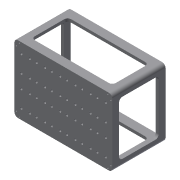
# Autodesk Inventor part: 05_Omniscope_base_v1
Saved by Autodesk Inventor 2019 (Build 230136000, 136)
## iProperties
Created: 2021-09-23
Part Number: 05_Omniscope_base_v1
Material: Generisch
Document SubType Name: Modeling
Designer: Muriel
Density: 1 g/cm^3
Appearance: Vorgabe
Author: Muriel
Autodesk Inventor part; units mm, degrees
(part 1 of 2)
ref_plane "YZ Plane" through (0, 0, 0) normal (1, 0, 0) x (0, 1, 0)
ref_plane "XZ Plane" through (0, 0, 0) normal (0, 1, 0) x (-1, 0, 0)
ref_plane "XY Plane" through (0, 0, 0) normal (0, 0, 1) x (1, 0, 0)
ref_plane "Arbeitsebene1" through (0, 0, 0) normal (0, 0, 1) x (1, 0, 0)
sketch "Skizze1" plane through (0, 0, 0) normal (0, 0, 1) x (1, 0, 0)
  arc A0 (4.5124, -17.9) -> (2.1124, -17.9) centre (3.3124, -16.3) ccw construction
  line L0 (4.5124, -17.9) -> (5.3124, -17.9) construction
  line L1 (5.3124, -17.9) -> (6.3124, -16.9) construction
  line L2 (6.3124, -16.9) -> (6.3124, 16.9) construction
  line L3 (6.3124, 16.9) -> (5.3124, 17.9) construction
  line L4 (5.3124, 17.9) -> (4.5124, 17.9) construction
  arc A1 (2.1124, 17.9) -> (4.5124, 17.9) centre (3.3124, 16.3) ccw construction
  line L5 (2.1124, 17.9) -> (-7.2876, 17.9) construction
  arc A2 (-9.6876, 17.9) -> (-7.2876, 17.9) centre (-8.4876, 16.3) ccw construction
  line L6 (-9.6876, 17.9) -> (-10.4876, 17.9) construction
  line L7 (-10.4876, 17.9) -> (-11.4876, 16.9) construction
  line L8 (-11.4876, 16.9) -> (-11.4876, -16.9) construction
  line L9 (-11.4876, -16.9) -> (-10.4876, -17.9) construction
  line L10 (-10.4876, -17.9) -> (-9.6876, -17.9) construction
  arc A3 (-7.2876, -17.9) -> (-9.6876, -17.9) centre (-8.4876, -16.3) ccw construction
  line L11 (-7.2876, -17.9) -> (2.1124, -17.9) construction
  circle A4 centre (-7.5876, -10) radius 2.45 construction
  circle A5 centre (2.4124, 10) radius 2.45 construction
  circle A6 centre (2.4124, -10) radius 2.45 construction
  circle A7 centre (-7.5876, 10) radius 2.45 construction
  line L12 (-5.4042, -5.4399) -> (-5.4042, -5.8455) construction
  line L13 (-5.4042, -5.8455) -> (-7.5626, -5.8455) construction
  line L14 (-7.5626, -5.8455) -> (-7.5626, -5.3491) construction
  spline S0 degree 2 poles (-7.5626, -5.3491) (-7.33, -5.1308) (-6.9159, -4.7252) (-6.7174, -4.5068) knots 0 0 0 1 2 2 2 construction
  spline S1 degree 2 poles (-6.7174, -4.5068) (-6.3174, -4.0671) (-6.0253, -3.5396) (-6.0253, -3.2588) knots 0 0 0 1 2 2 2 construction
  spline S2 degree 2 poles (-6.0253, -3.2588) (-6.0253, -3.1113) (-6.1161, -2.8901) (-6.1983, -2.8192) knots 0 0 0 1 2 2 2 construction
  spline S3 degree 2 poles (-6.1983, -2.8192) (-6.2806, -2.7483) (-6.4961, -2.6774) (-6.6266, -2.6774) knots 0 0 0 1 2 2 2 construction
  spline S4 degree 2 poles (-6.6266, -2.6774) (-6.7514, -2.6774) (-7.0067, -2.7397) (-7.123, -2.788) knots 0 0 0 1 2 2 2 construction
  spline S5 degree 2 poles (-7.123, -2.788) (-7.2222, -2.8277) (-7.4066, -2.9411) (-7.4633, -2.9808) knots 0 0 0 1 2 2 2 construction
  line L15 (-7.4633, -2.9808) -> (-7.4888, -2.9808) construction
  line L16 (-7.4888, -2.9808) -> (-7.4888, -2.4816) construction
  spline S6 degree 2 poles (-7.4888, -2.4816) (-7.3442, -2.4107) (-6.8251, -2.2718) (-6.5926, -2.2718) knots 0 0 0 1 2 2 2 construction
  spline S7 degree 2 poles (-6.5926, -2.2718) (-6.1019, -2.2718) (-5.5488, -2.7908) (-5.5488, -3.2333) knots 0 0 0 1 2 2 2 construction
  spline S8 degree 2 poles (-5.5488, -3.2333) (-5.5488, -3.4403) (-5.6452, -3.7863) (-5.7303, -3.9338) knots 0 0 0 1 2 2 2 construction
  spline S9 degree 2 poles (-5.7303, -3.9338) (-5.8154, -4.087) (-6.0622, -4.3876) (-6.1983, -4.5323) knots 0 0 0 1 2 2 2 construction
  spline S10 degree 2 poles (-6.1983, -4.5323) (-6.4195, -4.7734) (-6.9613, -5.2896) (-7.123, -5.4399) knots 0 0 0 1 2 2 2 construction
  line L17 (-7.123, -5.4399) -> (-5.4042, -5.4399) construction
  line L18 (1.5472, -2.3689) -> (1.5472, -5.8689) construction
  line L19 (1.5472, -5.8689) -> (1.0253, -5.8689) construction
  line L20 (1.0253, -5.8689) -> (-0.5233, -2.8511) construction
  line L21 (-0.5233, -2.8511) -> (-0.5233, -5.8689) construction
  line L22 (-0.5233, -5.8689) -> (-0.9572, -5.8689) construction
  line L23 (-0.9572, -5.8689) -> (-0.9572, -2.3689) construction
  line L24 (-0.9572, -2.3689) -> (-0.2964, -2.3689) construction
  line L25 (-0.2964, -2.3689) -> (1.1133, -5.14) construction
  line L26 (1.1133, -5.14) -> (1.1133, -2.3689) construction
  line L27 (1.1133, -2.3689) -> (1.5472, -2.3689) construction
  line L28 (3.2085, 3.1097) -> (3.2085, 2.7523) construction
  line L29 (3.2085, 2.7523) -> (1.501, 2.7523) construction
  line L30 (1.501, 2.7523) -> (1.501, 3.1097) construction
  line L31 (1.501, 3.1097) -> (2.1364, 3.1097) construction
  line L32 (2.1364, 3.1097) -> (2.1364, 5.4553) construction
  line L33 (2.1364, 5.4553) -> (1.501, 5.4553) construction
  line L34 (1.501, 5.4553) -> (1.501, 5.7758) construction
  spline S11 degree 2 poles (1.501, 5.7758) (1.8612, 5.7758) (2.2016, 5.98) (2.2243, 6.2636) knots 0 0 0 1 2 2 2 construction
  line L35 (2.2243, 6.2636) -> (2.5873, 6.2636) construction
  line L36 (2.5873, 6.2636) -> (2.5873, 3.1097) construction
  line L37 (2.5873, 3.1097) -> (3.2085, 3.1097) construction
  line L38 (-5.0676, 6.369) -> (-4.5939, 6.369) construction
  line L39 (-4.5939, 6.369) -> (-5.7994, 2.869) construction
  line L40 (-5.7994, 2.869) -> (-6.3014, 2.869) construction
  line L41 (-6.3014, 2.869) -> (-7.5068, 6.369) construction
  line L42 (-7.5068, 6.369) -> (-7.0076, 6.369) construction
  line L43 (-7.0076, 6.369) -> (-6.0376, 3.4618) construction
  line L44 (-6.0376, 3.4618) -> (-5.0676, 6.369) construction
  spline S12 degree 2 poles (-8.0968, 4.8261) (-7.9238, 4.6956) (-7.7366, 4.2985) (-7.7366, 3.9809) knots 0 0 0 1 2 2 2 construction
  spline S13 degree 2 poles (-7.7366, 3.9809) (-7.7366, 3.7284) (-7.8982, 3.2973) (-8.0457, 3.1385) knots 0 0 0 1 2 2 2 construction
  spline S14 degree 2 poles (-8.0457, 3.1385) (-8.1932, 2.9796) (-8.6328, 2.7953) (-8.9051, 2.7953) knots 0 0 0 1 2 2 2 construction
  spline S15 degree 2 poles (-8.9051, 2.7953) (-9.1547, 2.7953) (-9.6426, 2.9059) (-9.8212, 2.9938) knots 0 0 0 1 2 2 2 construction
  line L45 (-9.8212, 2.9938) -> (-9.8212, 3.4902) construction
  line L46 (-9.8212, 3.4902) -> (-9.7872, 3.4902) construction
  spline S16 degree 2 poles (-9.7872, 3.4902) (-9.7333, 3.4505) (-9.5319, 3.3484) (-9.41, 3.303) knots 0 0 0 1 2 2 2 construction
  spline S17 degree 2 poles (-9.41, 3.303) (-9.271, 3.2548) (-9.0413, 3.2009) (-8.8966, 3.2009) knots 0 0 0 1 2 2 2 construction
  spline S18 degree 2 poles (-8.8966, 3.2009) (-8.7548, 3.2009) (-8.4882, 3.303) (-8.3917, 3.4136) knots 0 0 0 1 2 2 2 construction
  spline S19 degree 2 poles (-8.3917, 3.4136) (-8.3038, 3.5185) (-8.2131, 3.7965) (-8.2131, 3.9837) knots 0 0 0 1 2 2 2 construction
  spline S20 degree 2 poles (-8.2131, 3.9837) (-8.2131, 4.1709) (-8.3152, 4.4091) (-8.4116, 4.4886) knots 0 0 0 1 2 2 2 construction
  spline S21 degree 2 poles (-8.4116, 4.4886) (-8.5109, 4.5765) (-8.8058, 4.6502) (-8.9845, 4.6502) knots 0 0 0 1 2 2 2 construction
  spline S22 degree 2 poles (-8.9845, 4.6502) (-9.1774, 4.6502) (-9.5603, 4.5907) (-9.6766, 4.5651) knots 0 0 0 1 2 2 2 construction
  line L47 (-9.6766, 4.5651) -> (-9.6766, 6.369) construction
  line L48 (-9.6766, 6.369) -> (-7.7564, 6.369) construction
  line L49 (-7.7564, 6.369) -> (-7.7564, 5.9578) construction
  line L50 (-7.7564, 5.9578) -> (-9.2256, 5.9578) construction
  line L51 (-9.2256, 5.9578) -> (-9.2256, 5.0246) construction
  spline S23 degree 2 poles (-9.2256, 5.0246) (-9.1405, 5.036) (-8.976, 5.0445) (-8.908, 5.0445) knots 0 0 0 1 2 2 2 construction
  spline S24 degree 2 poles (-8.908, 5.0445) (-8.6385, 5.0445) (-8.267, 4.9565) (-8.0968, 4.8261) knots 0 0 0 1 2 2 2 construction
  line L52 (-0.2036, 2.7523) -> (-0.6687, 2.7523) construction
  line L53 (-0.6687, 2.7523) -> (-0.6687, 5.8382) construction
  line L54 (-0.6687, 5.8382) -> (-1.843, 5.8382) construction
  line L55 (-1.843, 5.8382) -> (-1.843, 6.2523) construction
  line L56 (-1.843, 6.2523) -> (0.9706, 6.2523) construction
  line L57 (0.9706, 6.2523) -> (0.9706, 5.8382) construction
  line L58 (0.9706, 5.8382) -> (-0.2036, 5.8382) construction
  line L59 (-0.2036, 5.8382) -> (-0.2036, 2.7523) construction
  spline S25 degree 2 poles (-2.0577, -5.8349) (-2.2307, -5.886) (-2.5087, -5.937) (-2.7044, -5.937) knots 0 0 0 1 2 2 2 construction
  spline S26 degree 2 poles (-2.7044, -5.937) (-3.076, -5.937) (-3.6914, -5.7101) (-3.9127, -5.4804) knots 0 0 0 1 2 2 2 construction
  spline S27 degree 2 poles (-3.9127, -5.4804) (-4.1339, -5.2478) (-4.3693, -4.5614) (-4.3693, -4.1161) knots 0 0 0 1 2 2 2 construction
  spline S28 degree 2 poles (-4.3693, -4.1161) (-4.3693, -3.6935) (-4.1311, -3.0241) (-3.9098, -2.7859) knots 0 0 0 1 2 2 2 construction
  spline S29 degree 2 poles (-3.9098, -2.7859) (-3.6971, -2.5561) (-3.0731, -2.3065) (-2.7016, -2.3065) knots 0 0 0 1 2 2 2 construction
  spline S30 degree 2 poles (-2.7016, -2.3065) (-2.5229, -2.3065) (-2.1995, -2.3576) (-2.052, -2.403) knots 0 0 0 1 2 2 2 construction
  spline S31 degree 2 poles (-2.052, -2.403) (-1.9329, -2.437) (-1.6436, -2.5618) (-1.5557, -2.6072) knots 0 0 0 1 2 2 2 construction
  line L60 (-1.5557, -2.6072) -> (-1.5557, -3.1688) construction
  line L61 (-1.5557, -3.1688) -> (-1.5954, -3.1688) construction
  spline S32 degree 2 poles (-1.5954, -3.1688) (-1.6833, -3.0922) (-1.8677, -2.9532) (-2.0379, -2.8738) knots 0 0 0 1 2 2 2 construction
  spline S33 degree 2 poles (-2.0379, -2.8738) (-2.1797, -2.8029) (-2.5456, -2.7093) (-2.7554, -2.7093) knots 0 0 0 1 2 2 2 construction
  spline S34 degree 2 poles (-2.7554, -2.7093) (-3.2603, -2.7093) (-3.8843, -3.4694) (-3.8843, -4.1019) knots 0 0 0 1 2 2 2 construction
  spline S35 degree 2 poles (-3.8843, -4.1019) (-3.8843, -4.4536) (-3.7198, -4.9812) (-3.5638, -5.1627) knots 0 0 0 1 2 2 2 construction
  spline S36 degree 2 poles (-3.5638, -5.1627) (-3.4135, -5.3442) (-2.988, -5.5343) (-2.7214, -5.5343) knots 0 0 0 1 2 2 2 construction
  spline S37 degree 2 poles (-2.7214, -5.5343) (-2.5257, -5.5343) (-2.1343, -5.4775) (-2.001, -5.4208) knots 0 0 0 1 2 2 2 construction
  line L62 (-2.001, -5.4208) -> (-2.001, -4.516) construction
  line L63 (-2.001, -4.516) -> (-2.8122, -4.516) construction
  line L64 (-2.8122, -4.516) -> (-2.8122, -4.1076) construction
  line L65 (-2.8122, -4.1076) -> (-1.5415, -4.1076) construction
  line L66 (-1.5415, -4.1076) -> (-1.5415, -5.6364) construction
  spline S38 degree 2 poles (-1.5415, -5.6364) (-1.6294, -5.6761) (-1.9301, -5.798) (-2.0577, -5.8349) knots 0 0 0 1 2 2 2 construction
  spline S39 degree 2 poles (4.307, -2.6469) (4.6445, -2.871) (5.016, -3.6112) (5.016, -4.1218) knots 0 0 0 1 2 2 2 construction
  spline S40 degree 2 poles (5.016, -4.1218) (5.016, -4.6011) (4.6275, -5.3726) (4.3013, -5.5881) knots 0 0 0 1 2 2 2 construction
  spline S41 degree 2 poles (4.3013, -5.5881) (4.0347, -5.7555) (3.4873, -5.8689) (3.0618, -5.8689) knots 0 0 0 1 2 2 2 construction
  line L67 (3.0618, -5.8689) -> (2.2563, -5.8689) construction
  line L68 (2.2563, -5.8689) -> (2.2563, -2.3689) construction
  line L69 (2.2563, -2.3689) -> (3.0533, -2.3689) construction
  spline S42 degree 2 poles (3.0533, -2.3689) (3.5468, -2.3689) (4.1084, -2.5164) (4.307, -2.6469) knots 0 0 0 1 2 2 2 construction
  line L70 (-8.9921, -5.8455) -> (-9.4572, -5.8455) construction
  line L71 (-9.4572, -5.8455) -> (-9.4572, -2.7596) construction
  line L72 (-9.4572, -2.7596) -> (-10.6315, -2.7596) construction
  line L73 (-10.6315, -2.7596) -> (-10.6315, -2.3455) construction
  line L74 (-10.6315, -2.3455) -> (-7.8178, -2.3455) construction
  line L75 (-7.8178, -2.3455) -> (-7.8178, -2.7596) construction
  line L76 (-7.8178, -2.7596) -> (-8.9921, -2.7596) construction
  line L77 (-8.9921, -2.7596) -> (-8.9921, -5.8455) construction
  arc A8 (4.5124, -53.9) -> (2.1124, -53.9) centre (3.3124, -52.3) ccw construction
  line L78 (4.5124, -53.9) -> (5.3124, -53.9) construction
  line L79 (5.3124, -53.9) -> (6.3124, -52.9) construction
  line L80 (6.3124, -52.9) -> (6.3124, -19.1) construction
  line L81 (6.3124, -19.1) -> (5.3124, -18.1) construction
  line L82 (5.3124, -18.1) -> (4.5124, -18.1) construction
  arc A9 (2.1124, -18.1) -> (4.5124, -18.1) centre (3.3124, -19.7) ccw construction
  line L83 (2.1124, -18.1) -> (-7.2876, -18.1) construction
  arc A10 (-9.6876, -18.1) -> (-7.2876, -18.1) centre (-8.4876, -19.7) ccw construction
  line L84 (-9.6876, -18.1) -> (-10.4876, -18.1) construction
  line L85 (-10.4876, -18.1) -> (-11.4876, -19.1) construction
  line L86 (-11.4876, -19.1) -> (-11.4876, -52.9) construction
  line L87 (-11.4876, -52.9) -> (-10.4876, -53.9) construction
  line L88 (-10.4876, -53.9) -> (-9.6876, -53.9) construction
  arc A11 (-7.2876, -53.9) -> (-9.6876, -53.9) centre (-8.4876, -52.3) ccw construction
  line L89 (-7.2876, -53.9) -> (2.1124, -53.9) construction
  circle A12 centre (-7.5876, -46) radius 2.45 construction
  circle A13 centre (2.4124, -26) radius 2.45 construction
  circle A14 centre (2.4124, -46) radius 2.45 construction
  circle A15 centre (-7.5876, -26) radius 2.45 construction
  line L90 (-5.4042, -41.4399) -> (-5.4042, -41.8455) construction
  line L91 (-5.4042, -41.8455) -> (-7.5626, -41.8455) construction
  line L92 (-7.5626, -41.8455) -> (-7.5626, -41.3491) construction
  spline S43 degree 2 poles (-7.5626, -41.3491) (-7.33, -41.1308) (-6.9159, -40.7252) (-6.7174, -40.5068) knots 0 0 0 1 2 2 2 construction
  spline S44 degree 2 poles (-6.7174, -40.5068) (-6.3174, -40.0671) (-6.0253, -39.5396) (-6.0253, -39.2588) knots 0 0 0 1 2 2 2 construction
  spline S45 degree 2 poles (-6.0253, -39.2588) (-6.0253, -39.1113) (-6.1161, -38.8901) (-6.1983, -38.8192) knots 0 0 0 1 2 2 2 construction
  spline S46 degree 2 poles (-6.1983, -38.8192) (-6.2806, -38.7483) (-6.4961, -38.6774) (-6.6266, -38.6774) knots 0 0 0 1 2 2 2 construction
  spline S47 degree 2 poles (-6.6266, -38.6774) (-6.7514, -38.6774) (-7.0067, -38.7397) (-7.123, -38.788) knots 0 0 0 1 2 2 2 construction
  spline S48 degree 2 poles (-7.123, -38.788) (-7.2222, -38.8277) (-7.4066, -38.9411) (-7.4633, -38.9808) knots 0 0 0 1 2 2 2 construction
  line L93 (-7.4633, -38.9808) -> (-7.4888, -38.9808) construction
  line L94 (-7.4888, -38.9808) -> (-7.4888, -38.4816) construction
  spline S49 degree 2 poles (-7.4888, -38.4816) (-7.3442, -38.4107) (-6.8251, -38.2718) (-6.5926, -38.2718) knots 0 0 0 1 2 2 2 construction
  spline S50 degree 2 poles (-6.5926, -38.2718) (-6.1019, -38.2718) (-5.5488, -38.7908) (-5.5488, -39.2333) knots 0 0 0 1 2 2 2 construction
  spline S51 degree 2 poles (-5.5488, -39.2333) (-5.5488, -39.4403) (-5.6452, -39.7863) (-5.7303, -39.9338) knots 0 0 0 1 2 2 2 construction
  spline S52 degree 2 poles (-5.7303, -39.9338) (-5.8154, -40.087) (-6.0622, -40.3876) (-6.1983, -40.5323) knots 0 0 0 1 2 2 2 construction
  spline S53 degree 2 poles (-6.1983, -40.5323) (-6.4195, -40.7734) (-6.9613, -41.2896) (-7.123, -41.4399) knots 0 0 0 1 2 2 2 construction
  line L95 (-7.123, -41.4399) -> (-5.4042, -41.4399) construction
  line L96 (1.5472, -38.3689) -> (1.5472, -41.8689) construction
  line L97 (1.5472, -41.8689) -> (1.0253, -41.8689) construction
  line L98 (1.0253, -41.8689) -> (-0.5233, -38.8511) construction
  line L99 (-0.5233, -38.8511) -> (-0.5233, -41.8689) construction
  line L100 (-0.5233, -41.8689) -> (-0.9572, -41.8689) construction
  line L101 (-0.9572, -41.8689) -> (-0.9572, -38.3689) construction
  line L102 (-0.9572, -38.3689) -> (-0.2964, -38.3689) construction
  line L103 (-0.2964, -38.3689) -> (1.1133, -41.14) construction
  line L104 (1.1133, -41.14) -> (1.1133, -38.3689) construction
  line L105 (1.1133, -38.3689) -> (1.5472, -38.3689) construction
  line L106 (3.2085, -32.8903) -> (3.2085, -33.2477) construction
  line L107 (3.2085, -33.2477) -> (1.501, -33.2477) construction
  line L108 (1.501, -33.2477) -> (1.501, -32.8903) construction
  line L109 (1.501, -32.8903) -> (2.1364, -32.8903) construction
  line L110 (2.1364, -32.8903) -> (2.1364, -30.5447) construction
  line L111 (2.1364, -30.5447) -> (1.501, -30.5447) construction
  line L112 (1.501, -30.5447) -> (1.501, -30.2242) construction
  spline S54 degree 2 poles (1.501, -30.2242) (1.8612, -30.2242) (2.2016, -30.02) (2.2243, -29.7364) knots 0 0 0 1 2 2 2 construction
  line L113 (2.2243, -29.7364) -> (2.5873, -29.7364) construction
  line L114 (2.5873, -29.7364) -> (2.5873, -32.8903) construction
  line L115 (2.5873, -32.8903) -> (3.2085, -32.8903) construction
  line L116 (-5.0676, -29.631) -> (-4.5939, -29.631) construction
  line L117 (-4.5939, -29.631) -> (-5.7994, -33.131) construction
  line L118 (-5.7994, -33.131) -> (-6.3014, -33.131) construction
  line L119 (-6.3014, -33.131) -> (-7.5068, -29.631) construction
  line L120 (-7.5068, -29.631) -> (-7.0076, -29.631) construction
  line L121 (-7.0076, -29.631) -> (-6.0376, -32.5382) construction
  line L122 (-6.0376, -32.5382) -> (-5.0676, -29.631) construction
  spline S55 degree 2 poles (-8.0968, -31.1739) (-7.9238, -31.3044) (-7.7366, -31.7015) (-7.7366, -32.0191) knots 0 0 0 1 2 2 2 construction
  spline S56 degree 2 poles (-7.7366, -32.0191) (-7.7366, -32.2716) (-7.8982, -32.7027) (-8.0457, -32.8615) knots 0 0 0 1 2 2 2 construction
  spline S57 degree 2 poles (-8.0457, -32.8615) (-8.1932, -33.0204) (-8.6328, -33.2047) (-8.9051, -33.2047) knots 0 0 0 1 2 2 2 construction
  spline S58 degree 2 poles (-8.9051, -33.2047) (-9.1547, -33.2047) (-9.6426, -33.0941) (-9.8212, -33.0062) knots 0 0 0 1 2 2 2 construction
  line L123 (-9.8212, -33.0062) -> (-9.8212, -32.5098) construction
  line L124 (-9.8212, -32.5098) -> (-9.7872, -32.5098) construction
  spline S59 degree 2 poles (-9.7872, -32.5098) (-9.7333, -32.5495) (-9.5319, -32.6516) (-9.41, -32.697) knots 0 0 0 1 2 2 2 construction
  spline S60 degree 2 poles (-9.41, -32.697) (-9.271, -32.7452) (-9.0413, -32.7991) (-8.8966, -32.7991) knots 0 0 0 1 2 2 2 construction
  spline S61 degree 2 poles (-8.8966, -32.7991) (-8.7548, -32.7991) (-8.4882, -32.697) (-8.3917, -32.5864) knots 0 0 0 1 2 2 2 construction
  spline S62 degree 2 poles (-8.3917, -32.5864) (-8.3038, -32.4815) (-8.2131, -32.2035) (-8.2131, -32.0163) knots 0 0 0 1 2 2 2 construction
  spline S63 degree 2 poles (-8.2131, -32.0163) (-8.2131, -31.8291) (-8.3152, -31.5909) (-8.4116, -31.5114) knots 0 0 0 1 2 2 2 construction
  spline S64 degree 2 poles (-8.4116, -31.5114) (-8.5109, -31.4235) (-8.8058, -31.3498) (-8.9845, -31.3498) knots 0 0 0 1 2 2 2 construction
  spline S65 degree 2 poles (-8.9845, -31.3498) (-9.1774, -31.3498) (-9.5603, -31.4093) (-9.6766, -31.4349) knots 0 0 0 1 2 2 2 construction
  line L125 (-9.6766, -31.4349) -> (-9.6766, -29.631) construction
  line L126 (-9.6766, -29.631) -> (-7.7564, -29.631) construction
  line L127 (-7.7564, -29.631) -> (-7.7564, -30.0422) construction
  line L128 (-7.7564, -30.0422) -> (-9.2256, -30.0422) construction
  line L129 (-9.2256, -30.0422) -> (-9.2256, -30.9754) construction
  spline S66 degree 2 poles (-9.2256, -30.9754) (-9.1405, -30.964) (-8.976, -30.9555) (-8.908, -30.9555) knots 0 0 0 1 2 2 2 construction
  spline S67 degree 2 poles (-8.908, -30.9555) (-8.6385, -30.9555) (-8.267, -31.0435) (-8.0968, -31.1739) knots 0 0 0 1 2 2 2 construction
  line L130 (-0.2036, -33.2477) -> (-0.6687, -33.2477) construction
  line L131 (-0.6687, -33.2477) -> (-0.6687, -30.1618) construction
  line L132 (-0.6687, -30.1618) -> (-1.843, -30.1618) construction
  line L133 (-1.843, -30.1618) -> (-1.843, -29.7477) construction
  line L134 (-1.843, -29.7477) -> (0.9706, -29.7477) construction
  line L135 (0.9706, -29.7477) -> (0.9706, -30.1618) construction
  line L136 (0.9706, -30.1618) -> (-0.2036, -30.1618) construction
  line L137 (-0.2036, -30.1618) -> (-0.2036, -33.2477) construction
  spline S68 degree 2 poles (-2.0577, -41.8349) (-2.2307, -41.886) (-2.5087, -41.937) (-2.7044, -41.937) knots 0 0 0 1 2 2 2 construction
  spline S69 degree 2 poles (-2.7044, -41.937) (-3.076, -41.937) (-3.6914, -41.7101) (-3.9127, -41.4804) knots 0 0 0 1 2 2 2 construction
  spline S70 degree 2 poles (-3.9127, -41.4804) (-4.1339, -41.2478) (-4.3693, -40.5614) (-4.3693, -40.1161) knots 0 0 0 1 2 2 2 construction
  spline S71 degree 2 poles (-4.3693, -40.1161) (-4.3693, -39.6935) (-4.1311, -39.0241) (-3.9098, -38.7859) knots 0 0 0 1 2 2 2 construction
  spline S72 degree 2 poles (-3.9098, -38.7859) (-3.6971, -38.5561) (-3.0731, -38.3065) (-2.7016, -38.3065) knots 0 0 0 1 2 2 2 construction
  spline S73 degree 2 poles (-2.7016, -38.3065) (-2.5229, -38.3065) (-2.1995, -38.3576) (-2.052, -38.403) knots 0 0 0 1 2 2 2 construction
  spline S74 degree 2 poles (-2.052, -38.403) (-1.9329, -38.437) (-1.6436, -38.5618) (-1.5557, -38.6072) knots 0 0 0 1 2 2 2 construction
  line L138 (-1.5557, -38.6072) -> (-1.5557, -39.1688) construction
  line L139 (-1.5557, -39.1688) -> (-1.5954, -39.1688) construction
  spline S75 degree 2 poles (-1.5954, -39.1688) (-1.6833, -39.0922) (-1.8677, -38.9532) (-2.0379, -38.8738) knots 0 0 0 1 2 2 2 construction
  spline S76 degree 2 poles (-2.0379, -38.8738) (-2.1797, -38.8029) (-2.5456, -38.7093) (-2.7554, -38.7093) knots 0 0 0 1 2 2 2 construction
  spline S77 degree 2 poles (-2.7554, -38.7093) (-3.2603, -38.7093) (-3.8843, -39.4694) (-3.8843, -40.1019) knots 0 0 0 1 2 2 2 construction
  spline S78 degree 2 poles (-3.8843, -40.1019) (-3.8843, -40.4536) (-3.7198, -40.9812) (-3.5638, -41.1627) knots 0 0 0 1 2 2 2 construction
  spline S79 degree 2 poles (-3.5638, -41.1627) (-3.4135, -41.3442) (-2.988, -41.5343) (-2.7214, -41.5343) knots 0 0 0 1 2 2 2 construction
  spline S80 degree 2 poles (-2.7214, -41.5343) (-2.5257, -41.5343) (-2.1343, -41.4775) (-2.001, -41.4208) knots 0 0 0 1 2 2 2 construction
  line L140 (-2.001, -41.4208) -> (-2.001, -40.516) construction
  line L141 (-2.001, -40.516) -> (-2.8122, -40.516) construction
  line L142 (-2.8122, -40.516) -> (-2.8122, -40.1076) construction
  line L143 (-2.8122, -40.1076) -> (-1.5415, -40.1076) construction
  line L144 (-1.5415, -40.1076) -> (-1.5415, -41.6364) construction
  spline S81 degree 2 poles (-1.5415, -41.6364) (-1.6294, -41.6761) (-1.9301, -41.798) (-2.0577, -41.8349) knots 0 0 0 1 2 2 2 construction
  spline S82 degree 2 poles (4.307, -38.6469) (4.6445, -38.871) (5.016, -39.6112) (5.016, -40.1218) knots 0 0 0 1 2 2 2 construction
  spline S83 degree 2 poles (5.016, -40.1218) (5.016, -40.6011) (4.6275, -41.3726) (4.3013, -41.5881) knots 0 0 0 1 2 2 2 construction
  spline S84 degree 2 poles (4.3013, -41.5881) (4.0347, -41.7555) (3.4873, -41.8689) (3.0618, -41.8689) knots 0 0 0 1 2 2 2 construction
  line L145 (3.0618, -41.8689) -> (2.2563, -41.8689) construction
  line L146 (2.2563, -41.8689) -> (2.2563, -38.3689) construction
  line L147 (2.2563, -38.3689) -> (3.0533, -38.3689) construction
  spline S85 degree 2 poles (3.0533, -38.3689) (3.5468, -38.3689) (4.1084, -38.5164) (4.307, -38.6469) knots 0 0 0 1 2 2 2 construction
  line L148 (-8.9921, -41.8455) -> (-9.4572, -41.8455) construction
  line L149 (-9.4572, -41.8455) -> (-9.4572, -38.7596) construction
  line L150 (-9.4572, -38.7596) -> (-10.6315, -38.7596) construction
  line L151 (-10.6315, -38.7596) -> (-10.6315, -38.3455) construction
  line L152 (-10.6315, -38.3455) -> (-7.8178, -38.3455) construction
  line L153 (-7.8178, -38.3455) -> (-7.8178, -38.7596) construction
  line L154 (-7.8178, -38.7596) -> (-8.9921, -38.7596) construction
  line L155 (-8.9921, -38.7596) -> (-8.9921, -41.8455) construction
  arc A16 (94.5124, -53.9) -> (92.1124, -53.9) centre (93.3124, -52.3) ccw construction
  line L156 (94.5124, -53.9) -> (95.3124, -53.9) construction
  line L157 (95.3124, -53.9) -> (96.3124, -52.9) construction
  line L158 (96.3124, -52.9) -> (96.3124, -19.1) construction
  line L159 (96.3124, -19.1) -> (95.3124, -18.1) construction
  line L160 (95.3124, -18.1) -> (94.5124, -18.1) construction
  arc A17 (92.1124, -18.1) -> (94.5124, -18.1) centre (93.3124, -19.7) ccw construction
  line L161 (92.1124, -18.1) -> (82.7124, -18.1) construction
  arc A18 (80.3124, -18.1) -> (82.7124, -18.1) centre (81.5124, -19.7) ccw construction
  line L162 (80.3124, -18.1) -> (79.5124, -18.1) construction
  line L163 (79.5124, -18.1) -> (78.5124, -19.1) construction
  line L164 (78.5124, -19.1) -> (78.5124, -52.9) construction
  line L165 (78.5124, -52.9) -> (79.5124, -53.9) construction
  line L166 (79.5124, -53.9) -> (80.3124, -53.9) construction
  arc A19 (82.7124, -53.9) -> (80.3124, -53.9) centre (81.5124, -52.3) ccw construction
  line L167 (82.7124, -53.9) -> (92.1124, -53.9) construction
  circle A20 centre (82.4124, -46) radius 2.45 construction
  circle A21 centre (92.4124, -26) radius 2.45 construction
  circle A22 centre (92.4124, -46) radius 2.45 construction
  circle A23 centre (82.4124, -26) radius 2.45 construction
  line L168 (84.5958, -41.4399) -> (84.5958, -41.8455) construction
  line L169 (84.5958, -41.8455) -> (82.4374, -41.8455) construction
  line L170 (82.4374, -41.8455) -> (82.4374, -41.3491) construction
  spline S86 degree 2 poles (82.4374, -41.3491) (82.67, -41.1308) (83.0841, -40.7252) (83.2826, -40.5068) knots 0 0 0 1 2 2 2 construction
  spline S87 degree 2 poles (83.2826, -40.5068) (83.6826, -40.0671) (83.9747, -39.5396) (83.9747, -39.2588) knots 0 0 0 1 2 2 2 construction
  spline S88 degree 2 poles (83.9747, -39.2588) (83.9747, -39.1113) (83.8839, -38.8901) (83.8017, -38.8192) knots 0 0 0 1 2 2 2 construction
  spline S89 degree 2 poles (83.8017, -38.8192) (83.7194, -38.7483) (83.5039, -38.6774) (83.3734, -38.6774) knots 0 0 0 1 2 2 2 construction
  spline S90 degree 2 poles (83.3734, -38.6774) (83.2486, -38.6774) (82.9933, -38.7397) (82.877, -38.788) knots 0 0 0 1 2 2 2 construction
  spline S91 degree 2 poles (82.877, -38.788) (82.7778, -38.8277) (82.5934, -38.9411) (82.5367, -38.9808) knots 0 0 0 1 2 2 2 construction
  line L171 (82.5367, -38.9808) -> (82.5112, -38.9808) construction
  line L172 (82.5112, -38.9808) -> (82.5112, -38.4816) construction
  spline S92 degree 2 poles (82.5112, -38.4816) (82.6558, -38.4107) (83.1749, -38.2718) (83.4074, -38.2718) knots 0 0 0 1 2 2 2 construction
  spline S93 degree 2 poles (83.4074, -38.2718) (83.8981, -38.2718) (84.4512, -38.7908) (84.4512, -39.2333) knots 0 0 0 1 2 2 2 construction
  spline S94 degree 2 poles (84.4512, -39.2333) (84.4512, -39.4403) (84.3548, -39.7863) (84.2697, -39.9338) knots 0 0 0 1 2 2 2 construction
  spline S95 degree 2 poles (84.2697, -39.9338) (84.1846, -40.087) (83.9378, -40.3876) (83.8017, -40.5323) knots 0 0 0 1 2 2 2 construction
  spline S96 degree 2 poles (83.8017, -40.5323) (83.5805, -40.7734) (83.0387, -41.2896) (82.877, -41.4399) knots 0 0 0 1 2 2 2 construction
  line L173 (82.877, -41.4399) -> (84.5958, -41.4399) construction
  line L174 (91.5472, -38.3689) -> (91.5472, -41.8689) construction
  line L175 (91.5472, -41.8689) -> (91.0253, -41.8689) construction
  line L176 (91.0253, -41.8689) -> (89.4767, -38.8511) construction
  line L177 (89.4767, -38.8511) -> (89.4767, -41.8689) construction
  line L178 (89.4767, -41.8689) -> (89.0428, -41.8689) construction
  line L179 (89.0428, -41.8689) -> (89.0428, -38.3689) construction
  line L180 (89.0428, -38.3689) -> (89.7036, -38.3689) construction
  line L181 (89.7036, -38.3689) -> (91.1133, -41.14) construction
  line L182 (91.1133, -41.14) -> (91.1133, -38.3689) construction
  line L183 (91.1133, -38.3689) -> (91.5472, -38.3689) construction
  line L184 (93.2085, -32.8903) -> (93.2085, -33.2477) construction
  line L185 (93.2085, -33.2477) -> (91.501, -33.2477) construction
  line L186 (91.501, -33.2477) -> (91.501, -32.8903) construction
  line L187 (91.501, -32.8903) -> (92.1364, -32.8903) construction
  line L188 (92.1364, -32.8903) -> (92.1364, -30.5447) construction
  line L189 (92.1364, -30.5447) -> (91.501, -30.5447) construction
  line L190 (91.501, -30.5447) -> (91.501, -30.2242) construction
  spline S97 degree 2 poles (91.501, -30.2242) (91.8612, -30.2242) (92.2016, -30.02) (92.2243, -29.7364) knots 0 0 0 1 2 2 2 construction
  line L191 (92.2243, -29.7364) -> (92.5873, -29.7364) construction
  line L192 (92.5873, -29.7364) -> (92.5873, -32.8903) construction
  line L193 (92.5873, -32.8903) -> (93.2085, -32.8903) construction
  line L194 (84.9324, -29.631) -> (85.4061, -29.631) construction
  line L195 (85.4061, -29.631) -> (84.2006, -33.131) construction
  line L196 (84.2006, -33.131) -> (83.6986, -33.131) construction
  line L197 (83.6986, -33.131) -> (82.4932, -29.631) construction
  line L198 (82.4932, -29.631) -> (82.9924, -29.631) construction
  line L199 (82.9924, -29.631) -> (83.9624, -32.5382) construction
  line L200 (83.9624, -32.5382) -> (84.9324, -29.631) construction
  spline S98 degree 2 poles (81.9032, -31.1739) (82.0762, -31.3044) (82.2634, -31.7015) (82.2634, -32.0191) knots 0 0 0 1 2 2 2 construction
  spline S99 degree 2 poles (82.2634, -32.0191) (82.2634, -32.2716) (82.1018, -32.7027) (81.9543, -32.8615) knots 0 0 0 1 2 2 2 construction
  spline S100 degree 2 poles (81.9543, -32.8615) (81.8068, -33.0204) (81.3672, -33.2047) (81.0949, -33.2047) knots 0 0 0 1 2 2 2 construction
  spline S101 degree 2 poles (81.0949, -33.2047) (80.8453, -33.2047) (80.3574, -33.0941) (80.1788, -33.0062) knots 0 0 0 1 2 2 2 construction
  line L201 (80.1788, -33.0062) -> (80.1788, -32.5098) construction
  line L202 (80.1788, -32.5098) -> (80.2128, -32.5098) construction
  spline S102 degree 2 poles (80.2128, -32.5098) (80.2667, -32.5495) (80.4681, -32.6516) (80.59, -32.697) knots 0 0 0 1 2 2 2 construction
  spline S103 degree 2 poles (80.59, -32.697) (80.729, -32.7452) (80.9587, -32.7991) (81.1034, -32.7991) knots 0 0 0 1 2 2 2 construction
  spline S104 degree 2 poles (81.1034, -32.7991) (81.2452, -32.7991) (81.5118, -32.697) (81.6083, -32.5864) knots 0 0 0 1 2 2 2 construction
  spline S105 degree 2 poles (81.6083, -32.5864) (81.6962, -32.4815) (81.7869, -32.2035) (81.7869, -32.0163) knots 0 0 0 1 2 2 2 construction
  spline S106 degree 2 poles (81.7869, -32.0163) (81.7869, -31.8291) (81.6848, -31.5909) (81.5884, -31.5114) knots 0 0 0 1 2 2 2 construction
  spline S107 degree 2 poles (81.5884, -31.5114) (81.4891, -31.4235) (81.1942, -31.3498) (81.0155, -31.3498) knots 0 0 0 1 2 2 2 construction
  spline S108 degree 2 poles (81.0155, -31.3498) (80.8226, -31.3498) (80.4397, -31.4093) (80.3234, -31.4349) knots 0 0 0 1 2 2 2 construction
  line L203 (80.3234, -31.4349) -> (80.3234, -29.631) construction
  line L204 (80.3234, -29.631) -> (82.2436, -29.631) construction
  line L205 (82.2436, -29.631) -> (82.2436, -30.0422) construction
  line L206 (82.2436, -30.0422) -> (80.7744, -30.0422) construction
  line L207 (80.7744, -30.0422) -> (80.7744, -30.9754) construction
  spline S109 degree 2 poles (80.7744, -30.9754) (80.8595, -30.964) (81.024, -30.9555) (81.092, -30.9555) knots 0 0 0 1 2 2 2 construction
  spline S110 degree 2 poles (81.092, -30.9555) (81.3615, -30.9555) (81.733, -31.0435) (81.9032, -31.1739) knots 0 0 0 1 2 2 2 construction
  line L208 (89.7964, -33.2477) -> (89.3313, -33.2477) construction
  line L209 (89.3313, -33.2477) -> (89.3313, -30.1618) construction
  line L210 (89.3313, -30.1618) -> (88.157, -30.1618) construction
  line L211 (88.157, -30.1618) -> (88.157, -29.7477) construction
  line L212 (88.157, -29.7477) -> (90.9706, -29.7477) construction
  line L213 (90.9706, -29.7477) -> (90.9706, -30.1618) construction
  line L214 (90.9706, -30.1618) -> (89.7964, -30.1618) construction
  line L215 (89.7964, -30.1618) -> (89.7964, -33.2477) construction
  spline S111 degree 2 poles (87.9423, -41.8349) (87.7693, -41.886) (87.4913, -41.937) (87.2956, -41.937) knots 0 0 0 1 2 2 2 construction
  spline S112 degree 2 poles (87.2956, -41.937) (86.924, -41.937) (86.3086, -41.7101) (86.0873, -41.4804) knots 0 0 0 1 2 2 2 construction
  spline S113 degree 2 poles (86.0873, -41.4804) (85.8661, -41.2478) (85.6307, -40.5614) (85.6307, -40.1161) knots 0 0 0 1 2 2 2 construction
  spline S114 degree 2 poles (85.6307, -40.1161) (85.6307, -39.6935) (85.8689, -39.0241) (86.0902, -38.7859) knots 0 0 0 1 2 2 2 construction
  spline S115 degree 2 poles (86.0902, -38.7859) (86.3029, -38.5561) (86.9269, -38.3065) (87.2984, -38.3065) knots 0 0 0 1 2 2 2 construction
  spline S116 degree 2 poles (87.2984, -38.3065) (87.4771, -38.3065) (87.8005, -38.3576) (87.948, -38.403) knots 0 0 0 1 2 2 2 construction
  spline S117 degree 2 poles (87.948, -38.403) (88.0671, -38.437) (88.3564, -38.5618) (88.4443, -38.6072) knots 0 0 0 1 2 2 2 construction
  line L216 (88.4443, -38.6072) -> (88.4443, -39.1688) construction
  line L217 (88.4443, -39.1688) -> (88.4046, -39.1688) construction
  spline S118 degree 2 poles (88.4046, -39.1688) (88.3167, -39.0922) (88.1323, -38.9532) (87.9621, -38.8738) knots 0 0 0 1 2 2 2 construction
  spline S119 degree 2 poles (87.9621, -38.8738) (87.8203, -38.8029) (87.4544, -38.7093) (87.2446, -38.7093) knots 0 0 0 1 2 2 2 construction
  spline S120 degree 2 poles (87.2446, -38.7093) (86.7397, -38.7093) (86.1157, -39.4694) (86.1157, -40.1019) knots 0 0 0 1 2 2 2 construction
  spline S121 degree 2 poles (86.1157, -40.1019) (86.1157, -40.4536) (86.2802, -40.9812) (86.4362, -41.1627) knots 0 0 0 1 2 2 2 construction
  spline S122 degree 2 poles (86.4362, -41.1627) (86.5865, -41.3442) (87.012, -41.5343) (87.2786, -41.5343) knots 0 0 0 1 2 2 2 construction
  spline S123 degree 2 poles (87.2786, -41.5343) (87.4743, -41.5343) (87.8657, -41.4775) (87.999, -41.4208) knots 0 0 0 1 2 2 2 construction
  line L218 (87.999, -41.4208) -> (87.999, -40.516) construction
  line L219 (87.999, -40.516) -> (87.1878, -40.516) construction
  line L220 (87.1878, -40.516) -> (87.1878, -40.1076) construction
  line L221 (87.1878, -40.1076) -> (88.4585, -40.1076) construction
  line L222 (88.4585, -40.1076) -> (88.4585, -41.6364) construction
  spline S124 degree 2 poles (88.4585, -41.6364) (88.3706, -41.6761) (88.0699, -41.798) (87.9423, -41.8349) knots 0 0 0 1 2 2 2 construction
  spline S125 degree 2 poles (94.307, -38.6469) (94.6445, -38.871) (95.016, -39.6112) (95.016, -40.1218) knots 0 0 0 1 2 2 2 construction
  spline S126 degree 2 poles (95.016, -40.1218) (95.016, -40.6011) (94.6275, -41.3726) (94.3013, -41.5881) knots 0 0 0 1 2 2 2 construction
  spline S127 degree 2 poles (94.3013, -41.5881) (94.0347, -41.7555) (93.4873, -41.8689) (93.0618, -41.8689) knots 0 0 0 1 2 2 2 construction
  line L223 (93.0618, -41.8689) -> (92.2563, -41.8689) construction
  line L224 (92.2563, -41.8689) -> (92.2563, -38.3689) construction
  line L225 (92.2563, -38.3689) -> (93.0533, -38.3689) construction
  spline S128 degree 2 poles (93.0533, -38.3689) (93.5468, -38.3689) (94.1084, -38.5164) (94.307, -38.6469) knots 0 0 0 1 2 2 2 construction
  line L226 (81.0079, -41.8455) -> (80.5428, -41.8455) construction
  line L227 (80.5428, -41.8455) -> (80.5428, -38.7596) construction
  line L228 (80.5428, -38.7596) -> (79.3685, -38.7596) construction
  line L229 (79.3685, -38.7596) -> (79.3685, -38.3455) construction
  line L230 (79.3685, -38.3455) -> (82.1822, -38.3455) construction
  line L231 (82.1822, -38.3455) -> (82.1822, -38.7596) construction
  line L232 (82.1822, -38.7596) -> (81.0079, -38.7596) construction
  line L233 (81.0079, -38.7596) -> (81.0079, -41.8455) construction
  arc A24 (94.5124, -17.9) -> (92.1124, -17.9) centre (93.3124, -16.3) ccw construction
  line L234 (94.5124, -17.9) -> (95.3124, -17.9) construction
  line L235 (95.3124, -17.9) -> (96.3124, -16.9) construction
  line L236 (96.3124, -16.9) -> (96.3124, 16.9) construction
  line L237 (96.3124, 16.9) -> (95.3124, 17.9) construction
  line L238 (95.3124, 17.9) -> (94.5124, 17.9) construction
  arc A25 (92.1124, 17.9) -> (94.5124, 17.9) centre (93.3124, 16.3) ccw construction
  line L239 (92.1124, 17.9) -> (82.7124, 17.9) construction
  arc A26 (80.3124, 17.9) -> (82.7124, 17.9) centre (81.5124, 16.3) ccw construction
  line L240 (80.3124, 17.9) -> (79.5124, 17.9) construction
  line L241 (79.5124, 17.9) -> (78.5124, 16.9) construction
  line L242 (78.5124, 16.9) -> (78.5124, -16.9) construction
  line L243 (78.5124, -16.9) -> (79.5124, -17.9) construction
  line L244 (79.5124, -17.9) -> (80.3124, -17.9) construction
  arc A27 (82.7124, -17.9) -> (80.3124, -17.9) centre (81.5124, -16.3) ccw construction
  line L245 (82.7124, -17.9) -> (92.1124, -17.9) construction
  circle A28 centre (82.4124, -10) radius 2.45 construction
  circle A29 centre (92.4124, 10) radius 2.45 construction
  circle A30 centre (92.4124, -10) radius 2.45 construction
  circle A31 centre (82.4124, 10) radius 2.45 construction
  line L246 (84.5958, -5.4399) -> (84.5958, -5.8455) construction
  line L247 (84.5958, -5.8455) -> (82.4374, -5.8455) construction
  line L248 (82.4374, -5.8455) -> (82.4374, -5.3491) construction
  spline S129 degree 2 poles (82.4374, -5.3491) (82.67, -5.1308) (83.0841, -4.7252) (83.2826, -4.5068) knots 0 0 0 1 2 2 2 construction
  spline S130 degree 2 poles (83.2826, -4.5068) (83.6826, -4.0671) (83.9747, -3.5396) (83.9747, -3.2588) knots 0 0 0 1 2 2 2 construction
  spline S131 degree 2 poles (83.9747, -3.2588) (83.9747, -3.1113) (83.8839, -2.8901) (83.8017, -2.8192) knots 0 0 0 1 2 2 2 construction
  spline S132 degree 2 poles (83.8017, -2.8192) (83.7194, -2.7483) (83.5039, -2.6774) (83.3734, -2.6774) knots 0 0 0 1 2 2 2 construction
  spline S133 degree 2 poles (83.3734, -2.6774) (83.2486, -2.6774) (82.9933, -2.7397) (82.877, -2.788) knots 0 0 0 1 2 2 2 construction
  spline S134 degree 2 poles (82.877, -2.788) (82.7778, -2.8277) (82.5934, -2.9411) (82.5367, -2.9808) knots 0 0 0 1 2 2 2 construction
  line L249 (82.5367, -2.9808) -> (82.5112, -2.9808) construction
  line L250 (82.5112, -2.9808) -> (82.5112, -2.4816) construction
  spline S135 degree 2 poles (82.5112, -2.4816) (82.6558, -2.4107) (83.1749, -2.2718) (83.4074, -2.2718) knots 0 0 0 1 2 2 2 construction
  spline S136 degree 2 poles (83.4074, -2.2718) (83.8981, -2.2718) (84.4512, -2.7908) (84.4512, -3.2333) knots 0 0 0 1 2 2 2 construction
  spline S137 degree 2 poles (84.4512, -3.2333) (84.4512, -3.4403) (84.3548, -3.7863) (84.2697, -3.9338) knots 0 0 0 1 2 2 2 construction
  spline S138 degree 2 poles (84.2697, -3.9338) (84.1846, -4.087) (83.9378, -4.3876) (83.8017, -4.5323) knots 0 0 0 1 2 2 2 construction
  spline S139 degree 2 poles (83.8017, -4.5323) (83.5805, -4.7734) (83.0387, -5.2896) (82.877, -5.4399) knots 0 0 0 1 2 2 2 construction
  line L251 (82.877, -5.4399) -> (84.5958, -5.4399) construction
  line L252 (91.5472, -2.3689) -> (91.5472, -5.8689) construction
  line L253 (91.5472, -5.8689) -> (91.0253, -5.8689) construction
  line L254 (91.0253, -5.8689) -> (89.4767, -2.8511) construction
  line L255 (89.4767, -2.8511) -> (89.4767, -5.8689) construction
  line L256 (89.4767, -5.8689) -> (89.0428, -5.8689) construction
  line L257 (89.0428, -5.8689) -> (89.0428, -2.3689) construction
  line L258 (89.0428, -2.3689) -> (89.7036, -2.3689) construction
  line L259 (89.7036, -2.3689) -> (91.1133, -5.14) construction
  line L260 (91.1133, -5.14) -> (91.1133, -2.3689) construction
  line L261 (91.1133, -2.3689) -> (91.5472, -2.3689) construction
  line L262 (93.2085, 3.1097) -> (93.2085, 2.7523) construction
  line L263 (93.2085, 2.7523) -> (91.501, 2.7523) construction
  line L264 (91.501, 2.7523) -> (91.501, 3.1097) construction
  line L265 (91.501, 3.1097) -> (92.1364, 3.1097) construction
  line L266 (92.1364, 3.1097) -> (92.1364, 5.4553) construction
  line L267 (92.1364, 5.4553) -> (91.501, 5.4553) construction
  line L268 (91.501, 5.4553) -> (91.501, 5.7758) construction
  spline S140 degree 2 poles (91.501, 5.7758) (91.8612, 5.7758) (92.2016, 5.98) (92.2243, 6.2636) knots 0 0 0 1 2 2 2 construction
  line L269 (92.2243, 6.2636) -> (92.5873, 6.2636) construction
  line L270 (92.5873, 6.2636) -> (92.5873, 3.1097) construction
  line L271 (92.5873, 3.1097) -> (93.2085, 3.1097) construction
  line L272 (84.9324, 6.369) -> (85.4061, 6.369) construction
  line L273 (85.4061, 6.369) -> (84.2006, 2.869) construction
  line L274 (84.2006, 2.869) -> (83.6986, 2.869) construction
  line L275 (83.6986, 2.869) -> (82.4932, 6.369) construction
  line L276 (82.4932, 6.369) -> (82.9924, 6.369) construction
  line L277 (82.9924, 6.369) -> (83.9624, 3.4618) construction
  line L278 (83.9624, 3.4618) -> (84.9324, 6.369) construction
  spline S141 degree 2 poles (81.9032, 4.8261) (82.0762, 4.6956) (82.2634, 4.2985) (82.2634, 3.9809) knots 0 0 0 1 2 2 2 construction
  spline S142 degree 2 poles (82.2634, 3.9809) (82.2634, 3.7284) (82.1018, 3.2973) (81.9543, 3.1385) knots 0 0 0 1 2 2 2 construction
  spline S143 degree 2 poles (81.9543, 3.1385) (81.8068, 2.9796) (81.3672, 2.7953) (81.0949, 2.7953) knots 0 0 0 1 2 2 2 construction
  spline S144 degree 2 poles (81.0949, 2.7953) (80.8453, 2.7953) (80.3574, 2.9059) (80.1788, 2.9938) knots 0 0 0 1 2 2 2 construction
  line L279 (80.1788, 2.9938) -> (80.1788, 3.4902) construction
  line L280 (80.1788, 3.4902) -> (80.2128, 3.4902) construction
  spline S145 degree 2 poles (80.2128, 3.4902) (80.2667, 3.4505) (80.4681, 3.3484) (80.59, 3.303) knots 0 0 0 1 2 2 2 construction
  spline S146 degree 2 poles (80.59, 3.303) (80.729, 3.2548) (80.9587, 3.2009) (81.1034, 3.2009) knots 0 0 0 1 2 2 2 construction
  spline S147 degree 2 poles (81.1034, 3.2009) (81.2452, 3.2009) (81.5118, 3.303) (81.6083, 3.4136) knots 0 0 0 1 2 2 2 construction
  spline S148 degree 2 poles (81.6083, 3.4136) (81.6962, 3.5185) (81.7869, 3.7965) (81.7869, 3.9837) knots 0 0 0 1 2 2 2 construction
  spline S149 degree 2 poles (81.7869, 3.9837) (81.7869, 4.1709) (81.6848, 4.4091) (81.5884, 4.4886) knots 0 0 0 1 2 2 2 construction
  spline S150 degree 2 poles (81.5884, 4.4886) (81.4891, 4.5765) (81.1942, 4.6502) (81.0155, 4.6502) knots 0 0 0 1 2 2 2 construction
  spline S151 degree 2 poles (81.0155, 4.6502) (80.8226, 4.6502) (80.4397, 4.5907) (80.3234, 4.5651) knots 0 0 0 1 2 2 2 construction
  line L281 (80.3234, 4.5651) -> (80.3234, 6.369) construction
  line L282 (80.3234, 6.369) -> (82.2436, 6.369) construction
  line L283 (82.2436, 6.369) -> (82.2436, 5.9578) construction
  line L284 (82.2436, 5.9578) -> (80.7744, 5.9578) construction
  line L285 (80.7744, 5.9578) -> (80.7744, 5.0246) construction
  spline S152 degree 2 poles (80.7744, 5.0246) (80.8595, 5.036) (81.024, 5.0445) (81.092, 5.0445) knots 0 0 0 1 2 2 2 construction
  spline S153 degree 2 poles (81.092, 5.0445) (81.3615, 5.0445) (81.733, 4.9565) (81.9032, 4.8261) knots 0 0 0 1 2 2 2 construction
  line L286 (89.7964, 2.7523) -> (89.3313, 2.7523) construction
  line L287 (89.3313, 2.7523) -> (89.3313, 5.8382) construction
  line L288 (89.3313, 5.8382) -> (88.157, 5.8382) construction
  line L289 (88.157, 5.8382) -> (88.157, 6.2523) construction
  line L290 (88.157, 6.2523) -> (90.9706, 6.2523) construction
  line L291 (90.9706, 6.2523) -> (90.9706, 5.8382) construction
  line L292 (90.9706, 5.8382) -> (89.7964, 5.8382) construction
  line L293 (89.7964, 5.8382) -> (89.7964, 2.7523) construction
  spline S154 degree 2 poles (87.9423, -5.8349) (87.7693, -5.886) (87.4913, -5.937) (87.2956, -5.937) knots 0 0 0 1 2 2 2 construction
  spline S155 degree 2 poles (87.2956, -5.937) (86.924, -5.937) (86.3086, -5.7101) (86.0873, -5.4804) knots 0 0 0 1 2 2 2 construction
  spline S156 degree 2 poles (86.0873, -5.4804) (85.8661, -5.2478) (85.6307, -4.5614) (85.6307, -4.1161) knots 0 0 0 1 2 2 2 construction
  spline S157 degree 2 poles (85.6307, -4.1161) (85.6307, -3.6935) (85.8689, -3.0241) (86.0902, -2.7859) knots 0 0 0 1 2 2 2 construction
  spline S158 degree 2 poles (86.0902, -2.7859) (86.3029, -2.5561) (86.9269, -2.3065) (87.2984, -2.3065) knots 0 0 0 1 2 2 2 construction
  spline S159 degree 2 poles (87.2984, -2.3065) (87.4771, -2.3065) (87.8005, -2.3576) (87.948, -2.403) knots 0 0 0 1 2 2 2 construction
  spline S160 degree 2 poles (87.948, -2.403) (88.0671, -2.437) (88.3564, -2.5618) (88.4443, -2.6072) knots 0 0 0 1 2 2 2 construction
  line L294 (88.4443, -2.6072) -> (88.4443, -3.1688) construction
  line L295 (88.4443, -3.1688) -> (88.4046, -3.1688) construction
  spline S161 degree 2 poles (88.4046, -3.1688) (88.3167, -3.0922) (88.1323, -2.9532) (87.9621, -2.8738) knots 0 0 0 1 2 2 2 construction
  spline S162 degree 2 poles (87.9621, -2.8738) (87.8203, -2.8029) (87.4544, -2.7093) (87.2446, -2.7093) knots 0 0 0 1 2 2 2 construction
  spline S163 degree 2 poles (87.2446, -2.7093) (86.7397, -2.7093) (86.1157, -3.4694) (86.1157, -4.1019) knots 0 0 0 1 2 2 2 construction
  spline S164 degree 2 poles (86.1157, -4.1019) (86.1157, -4.4536) (86.2802, -4.9812) (86.4362, -5.1627) knots 0 0 0 1 2 2 2 construction
  spline S165 degree 2 poles (86.4362, -5.1627) (86.5865, -5.3442) (87.012, -5.5343) (87.2786, -5.5343) knots 0 0 0 1 2 2 2 construction
  spline S166 degree 2 poles (87.2786, -5.5343) (87.4743, -5.5343) (87.8657, -5.4775) (87.999, -5.4208) knots 0 0 0 1 2 2 2 construction
  line L296 (87.999, -5.4208) -> (87.999, -4.516) construction
  line L297 (87.999, -4.516) -> (87.1878, -4.516) construction
  line L298 (87.1878, -4.516) -> (87.1878, -4.1076) construction
  line L299 (87.1878, -4.1076) -> (88.4585, -4.1076) construction
  line L300 (88.4585, -4.1076) -> (88.4585, -5.6364) construction
  spline S167 degree 2 poles (88.4585, -5.6364) (88.3706, -5.6761) (88.0699, -5.798) (87.9423, -5.8349) knots 0 0 0 1 2 2 2 construction
  spline S168 degree 2 poles (94.307, -2.6469) (94.6445, -2.871) (95.016, -3.6112) (95.016, -4.1218) knots 0 0 0 1 2 2 2 construction
  spline S169 degree 2 poles (95.016, -4.1218) (95.016, -4.6011) (94.6275, -5.3726) (94.3013, -5.5881) knots 0 0 0 1 2 2 2 construction
  spline S170 degree 2 poles (94.3013, -5.5881) (94.0347, -5.7555) (93.4873, -5.8689) (93.0618, -5.8689) knots 0 0 0 1 2 2 2 construction
  line L301 (93.0618, -5.8689) -> (92.2563, -5.8689) construction
  line L302 (92.2563, -5.8689) -> (92.2563, -2.3689) construction
  line L303 (92.2563, -2.3689) -> (93.0533, -2.3689) construction
  spline S171 degree 2 poles (93.0533, -2.3689) (93.5468, -2.3689) (94.1084, -2.5164) (94.307, -2.6469) knots 0 0 0 1 2 2 2 construction
  line L304 (81.0079, -5.8455) -> (80.5428, -5.8455) construction
  line L305 (80.5428, -5.8455) -> (80.5428, -2.7596) construction
  line L306 (80.5428, -2.7596) -> (79.3685, -2.7596) construction
  line L307 (79.3685, -2.7596) -> (79.3685, -2.3455) construction
  line L308 (79.3685, -2.3455) -> (82.1822, -2.3455) construction
  line L309 (82.1822, -2.3455) -> (82.1822, -2.7596) construction
  line L310 (82.1822, -2.7596) -> (81.0079, -2.7596) construction
  line L311 (81.0079, -2.7596) -> (81.0079, -5.8455) construction
  line L312 (96.3476, 17.9352) -> (-11.5959, 17.9352)
  line L313 (-11.5959, 17.9352) -> (-11.5959, -53.9)
  line L314 (-11.5959, -53.9) -> (96.3476, -53.9)
  line L315 (96.3476, -53.9) -> (96.3476, 17.9352)
  line L316 (-15.5959, 21.9352) -> (100.3476, 21.9352)
  line L317 (100.3476, 21.9352) -> (100.3476, -57.9)
  line L318 (100.3476, -57.9) -> (-15.5959, -57.9)
  line L319 (-15.5959, -57.9) -> (-15.5959, 21.9352)
  point P0 (0, 0)
  dimension "d0" = 4
  constraints: 16 end point, 4 parallel, 2 perpendicular, 1 horizontal, 3 other
  measures "d0" distance between parallel lines of L312 L316
extrude "Extrusion1" add sketch "Skizze1" along normal blind 4 contours L315 L314 L313 L312 | L316 L317 L318 L319
sketch "Skizze2" plane through (0, 0, 0) normal (0, 0, -1) x (-1, 0, 0)
  circle A0 centre (-2.4124, -10) radius 0.5 projected
  circle A1 centre (7.5876, 10) radius 0.5 projected
  circle A2 centre (-2.4124, 10) radius 0.5 projected
  circle A3 centre (7.5876, -10) radius 0.5 projected
  circle A4 centre (-3.3124, -16.3) radius 0.9 projected
  circle A5 centre (8.4876, -16.3) radius 0.9 projected
  circle A6 centre (8.4876, 16.3) radius 0.9 projected
  circle A7 centre (-3.3124, 16.3) radius 0.9 projected
  line L0 (11.4876, 16.9) -> (11.4876, -16.9) projected
  line L1 (10.4876, 17.9) -> (11.4876, 16.9) projected
  line L2 (-5.3124, 17.9) -> (10.4876, 17.9) projected
  line L3 (-6.3124, 16.9) -> (-5.3124, 17.9) projected
  line L4 (-6.3124, -16.9) -> (-6.3124, 16.9) projected
  line L5 (-5.3124, -17.9) -> (-6.3124, -16.9) projected
  line L6 (10.4876, -17.9) -> (-5.3124, -17.9) projected
  line L7 (11.4876, -16.9) -> (10.4876, -17.9) projected
  point P0 (0, 0)
hole "Bohrung1" at (2.4124, -10, 0) at (-7.5876, -10, 0) at (2.4124, 10, 0) at (-7.5876, 10, 0) direction (0, 0, 1) diameter 2.8 depth 12 tip angle 118 counterbore diameter 6 counterbore depth 2
pattern_linear "Rechteckige Anordnung1" count 6 spacing 18 along (1, 0, 0) count 2 spacing 36 along (0, -1, 0) of "Bohrung1"